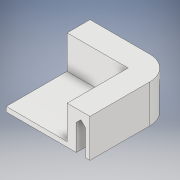
# Autodesk Inventor part: Corner Piece
Saved by Autodesk Inventor 2019 (Build 230136000, 136)
## iProperties
Created: 2019-02-08
Part Number: Corner Piece
Material: Generic
Document SubType Name: Modeling
Designer: scigu
Density: 1 g/cm^3
Appearance: White
Author: scigu
Autodesk Inventor part; units mm, degrees
ref_plane "YZ Plane" through (0, 0, 0) normal (1, 0, 0) x (0, 1, 0)
ref_plane "XZ Plane" through (0, 0, 0) normal (0, 1, 0) x (-1, 0, 0)
ref_plane "XY Plane" through (0, 0, 0) normal (0, 0, 1) x (1, 0, 0)
sketch "Sketch1" plane through (0, 0, 0) normal (0, 1, 0) x (-1, 0, 0)
  line L0 (0, 0) -> (-9.525, 0)
  line L1 (-9.525, 0) -> (-9.525, -9.525)
  line L2 (-9.525, -9.525) -> (0, -9.525)
  line L3 (0, -9.525) -> (0, 0)
  line L4 (0, 0) -> (25.4, 0)
  line L5 (25.4, 0) -> (25.4, -9.525)
  line L6 (25.4, -9.525) -> (0, -9.525)
  line L7 (0, -9.525) -> (0, 0)
  line L8 (0, 0) -> (-9.525, 0)
  line L9 (-9.525, 0) -> (-9.525, 25.4)
  line L10 (-9.525, 25.4) -> (0, 25.4)
  line L11 (0, 25.4) -> (0, 0)
  dimension "d0" = 9.525
  dimension "d1" = 9.525
  dimension "d2" = 25.4
  dimension "d3" = 9.525
  dimension "d4" = 9.525
  dimension "d5" = 25.4
  constraints: 24 end point, 6 parallel, 3 horizontal, 3 perpendicular
  measures "d0" distance of L2.end L1.end
  measures "d1" distance of L1.end L0.end
  measures "d2" distance of L5.end L6.end
  measures "d3" distance of L4.end L5.end
  measures "d4" distance of L9.end L10.end
  measures "d5" distance of L8.end L9.end
extrude "Extrusion1" add sketch "Sketch1" along normal blind 15.875
sketch "Sketch2" plane through (0, 0, 0) normal (0, -1, 0) x (1, 0, 0)
  line L0 (0, 0) -> (7.62, 0) construction
  line L1 (7.62, 0) -> (7.62, -7.62) construction
  line L2 (7.62, -7.62) -> (0, -7.62) construction
  line L3 (0, -7.62) -> (0, 0) construction
  line L4 (7.62, -7.62) -> (3.81, -7.62)
  line L5 (3.81, -7.62) -> (3.81, 25.4)
  line L6 (3.81, 25.4) -> (7.62, 25.4)
  line L7 (7.62, 25.4) -> (7.62, -7.62)
  line L8 (7.62, -7.62) -> (-25.4, -7.62)
  line L9 (-25.4, -7.62) -> (-25.4, -3.81)
  line L10 (-25.4, -3.81) -> (7.62, -3.81)
  line L11 (7.62, -3.81) -> (7.62, -7.62)
  dimension "d8" = 7.62
  dimension "d9" = 7.62
  dimension "d10" = 3.81
  dimension "d11" = 33.02
  dimension "d12" = 33.02
  dimension "d13" = 3.81
  constraints: 24 end point, 6 parallel, 3 horizontal, 3 perpendicular
  measures "d8" distance of L1.end L2.end
  measures "d9" distance of L0.end L1.end
  measures "d10" distance of L5.end L6.end
  measures "d11" distance of L4.end L5.end
  measures "d12" distance of L9.end L10.end
  measures "d13" distance of L8.end L9.end
extrude "Extrusion2" cut sketch "Sketch2" against normal blind 12.7
fillet "Fillet1" radius 10 1 edges at (9.525, 7.9375, -9.525)
chamfer "Chamfer1" distance 1.8415 angle 45 4 edges at (7.62, 12.7, 10.0019) (3.81, 12.7, 10.795) (-10.795, 12.7, -3.81) (-10.0019, 12.7, -7.62)
sketch "Sketch3" plane through (0, 0, 0) normal (0, -1, 0) x (1, 0, 0)
  line L0 (0, 0) -> (-25.4, 0)
  line L1 (-25.4, 0) -> (-25.4, 25.4)
  line L2 (-25.4, 25.4) -> (0, 25.4)
  line L3 (0, 25.4) -> (0, 0)
  dimension "d20" = 25.4
  dimension "d21" = 25.4
  constraints: 8 end point, 2 parallel, 1 horizontal, 1 perpendicular
  measures "d20" distance of L1.end L2.end
  measures "d21" distance of L0.end L1.end
extrude "Extrusion3" add sketch "Sketch3" against normal blind 2
body "Solid1"
